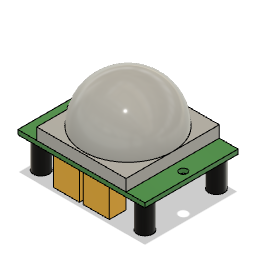
Dectecteur v4 (Autodesk Fusion 360 archive; units mm, degrees)
design "SEN0018_Detecteur UI.R"
Autodesk Fusion 360 part; units mm, degrees
sketch "Esquisse1" plane through (0, 0, 0) normal (0, 1, 0) x (1, 0, 0)
  line L0 (0, 0) -> (32.7, 0)
  line L1 (32.7, 0) -> (32.7, -24)
  line L2 (32.7, -24) -> (0, -24)
  line L3 (0, -24) -> (0, 0)
  dimension "d1" = 32.7
  dimension "d2" = 24
  constraint horizontal L0
  constraint vertical L1
  constraint horizontal L2
  constraint vertical L3
  constraint coincident L0.start L3.end
  measures "d1" distance of L0.start L0.end
  measures "d2" distance of L0.start L2.end
extrude "Extrusion1" add sketch "Esquisse1" along normal blind 1.15 makes body 1
sketch "Esquisse2" plane through (0, 1.15, 0) normal (0, 1, 0) x (-1, 0, 0)
  line L0 (0, 24) -> (-32.7, 24)
  line L1 (-32.7, 24) -> (-32.7, 0)
  line L2 (-32.7, 0) -> (0, 0)
  line L3 (0, 0) -> (0, 24)
  line L4 (-4.85, 0) -> (-27.85, 0)
  line L5 (-27.85, 0) -> (-27.85, 24)
  line L6 (-27.85, 24) -> (-4.85, 24)
  line L7 (-4.85, 24) -> (-4.85, 0)
  dimension "d5" = 23
  constraint horizontal L4
  constraint vertical L5
  constraint horizontal L6
  constraint vertical L7
  constraint coincident L0 L5.end
  constraint coincident L2 L4.start
  constraint midpoint L2 L4
  measures "d5" distance of L4.start L4.end
extrude "Extrusion2" add sketch "Esquisse2" along normal blind 3 separate body contours L0 L2 L4 L5 L6 L7 makes body 2
ref_plane "Plan de construction1" through (16.35, 2.65, 12) normal (0, 0, 1) x (1, 0, 0)
sketch "Esquisse3" plane through (16.35, 2.65, 12) normal (0, 0, 1) x (1, 0, 0)
  arc A0 (0, 13) -> (-11.5, 1.5) centre (0, 1.5) ccw
  line L0 (0, 1.5) -> (0, 13) construction
  line L1 (0, 1.5) -> (-11.5, 1.5) construction
  line L2 (-11.5, 1.5) -> (11.5, 1.5)
  line L3 (0, 13) -> (0, 1.5)
  point P0 (-11.5, 1.5)
  dimension "d8" = 90
  constraint coincident P0 A0.end
  constraint midpoint A0.centre L2
  constraint coincident A0.centre L0.start
  measures "d8" angle of L0 L1
revolve "Révolution1" add sketch "Esquisse3" angle 360 about axis through (16.35, 15.65, 12) along (0, -1, 0) bodies 2
sketch "Esquisse5" plane through (0, 0, 0) normal (0, -1, 0) x (1, 0, 0)
  line L0 (32.7, 24) -> (0, 24)
  line L1 (0, 24) -> (0, 0)
  line L2 (0, 0) -> (32.7, 0)
  line L3 (32.7, 0) -> (32.7, 24)
  circle A0 centre (3, 21) radius 2
  circle A1 centre (29.7, 21) radius 2
  circle A2 centre (29.7, 2.5849) radius 2
  circle A3 centre (3, 2.5849) radius 2
  line L4 (8.3, 23.15) -> (15, 23.15)
  line L5 (15, 23.15) -> (15, 18.85)
  line L6 (15, 18.85) -> (8.3, 18.85)
  line L7 (8.3, 18.85) -> (8.3, 23.15)
  line L8 (16, 23.15) -> (22.7, 23.15)
  line L9 (22.7, 23.15) -> (22.7, 18.85)
  line L10 (22.7, 18.85) -> (16, 18.85)
  line L11 (16, 18.85) -> (16, 23.15)
  line L12 (12.35, 3.7849) -> (20.35, 3.7849)
  line L13 (20.35, 3.7849) -> (20.35, 1.3849)
  line L14 (20.35, 1.3849) -> (12.35, 1.3849)
  line L15 (12.35, 1.3849) -> (12.35, 3.7849)
  line L16 (14.35, 2.8349) -> (14.85, 2.8349)
  line L17 (14.85, 2.8349) -> (14.85, 2.3349)
  line L18 (14.85, 2.3349) -> (14.35, 2.3349)
  line L19 (14.35, 2.3349) -> (14.35, 2.8349)
  line L20 (17.85, 2.8349) -> (18.35, 2.8349)
  line L21 (18.35, 2.8349) -> (18.35, 2.3349)
  line L22 (18.35, 2.3349) -> (17.85, 2.3349)
  line L23 (17.85, 2.3349) -> (17.85, 2.8349)
  line L24 (16.1, 2.8349) -> (16.6, 2.8349)
  line L25 (16.6, 2.8349) -> (16.6, 2.3349)
  line L26 (16.6, 2.3349) -> (16.1, 2.3349)
  line L27 (16.1, 2.3349) -> (16.1, 2.8349)
  line L28 (3, 21) -> (29.7, 21) construction
  line L29 (29.7, 21) -> (29.7, 2.5849) construction
  line L30 (29.7, 2.5849) -> (3, 2.5849) construction
  line L31 (3, 2.5849) -> (3, 21) construction
  line L32 (16.35, 2.3349) -> (16.35, 1.3849) construction
  line L33 (16.35, 1.3849) -> (16.35, 0) construction
  line L34 (18.35, 2.5849) -> (20.35, 2.5849) construction
  dimension "d10" = 4
  dimension "d11" = 4
  dimension "d12" = 4
  dimension "d13" = 4
  dimension "d14" = 3
  dimension "d15" = 3
  dimension "d16" = 3
  dimension "d17" = 2.5849
  dimension "d18" = 6.7
  dimension "d19" = 4.3
  dimension "d20" = 1
  dimension "d21" = 2.15
  dimension "d22" = 7
  dimension "d23" = 8
  dimension "d24" = 0.5
  dimension "d25" = 0.5
  dimension "d26" = 2
  dimension "d27" = 2
  dimension "d29" = 2.4
  constraint horizontal L4
  constraint vertical L5
  constraint horizontal L6
  constraint vertical L7
  constraint horizontal L8
  constraint vertical L9
  constraint horizontal L10
  constraint vertical L11
  constraint horizontal L12
  constraint vertical L13
  constraint horizontal L14
  constraint vertical L15
  constraint horizontal L16
  constraint vertical L17
  constraint horizontal L18
  constraint vertical L19
  constraint horizontal L20
  constraint vertical L21
  constraint horizontal L22
  constraint vertical L23
  constraint horizontal L24
  constraint vertical L25
  constraint horizontal L26
  constraint vertical L27
  constraint horizontal L28
  constraint vertical L29
  constraint horizontal L30
  constraint vertical L31
  constraint coincident A0.centre L28.start
  constraint coincident A1.centre L28.end
  constraint coincident A2.centre L29.end
  constraint coincident A3.centre L30.end
  constraint equal L6 L10
  constraint equal L5 L11
  constraint collinear L4 L8
  constraint equal L16 L20
  constraint equal L20 L23
  constraint equal L21 L27
  constraint equal L24 L27
  constraint collinear L16 L24
  constraint collinear L20 L24
  constraint midpoint L26 L32.start
  constraint coincident L14 L32.end
  constraint midpoint L14 L32.end
  constraint vertical L32
  constraint coincident L2 L33.end
  constraint midpoint L2 L33.end
  constraint vertical L33
  constraint midpoint L21 L34.start
  constraint midpoint L13 L34.end
  constraint horizontal L34
  constraint coincident L30 L34.end
  measures "d10" diameter of A0
  measures "d11" diameter of A1
  measures "d12" diameter of A2
  measures "d13" diameter of A3
  measures "d14" distance of L0 A0.centre
  measures "d15" distance of L1 A0.centre
  measures "d16" distance of L3 L29
  measures "d17" distance of L2 L30
  measures "d18" distance of L5.end L6.end
  measures "d19" distance of L4.start L6.end
  measures "d20" distance of L5 L11
  measures "d21" distance of L8 L28
  measures "d22" distance of A1.centre L9
  measures "d23" distance of L12.start L12.end
  measures "d24" distance of L16.start L16.end
  measures "d25" distance of L16.start L18.end
  measures "d26" distance of L15 L18.end
  measures "d27" distance of L13 L21.end
  measures "d29" distance of L12.end L13.end
extrude "Extrusion3" add sketch "Esquisse5" along normal blind 7.8 separate body contours A0 | A1 | A2 | A3 makes body 3 at (4.9901, -5.2, 2.3857) makes body 4 at (31.6901, -5.2, 20.8009) makes body 5 at (4.9901, -5.2, 20.8009) makes body 6 at (31.6901, -5.2, 2.3857)
extrude "Extrusion4" add sketch "Esquisse5" along normal blind 8 separate body contours L4 L5 L6 L7 | L8 L9 L10 L11 makes body 7 at (10.5333, -2.6667, 23.15) makes body 8 at (20.4667, -2.6667, 18.85)
extrude "Extrusion5" add sketch "Esquisse5" along normal blind 8.3 separate body contours L16 L17 L18 L19 | L20 L21 L22 L23 | L24 L25 L26 L27 makes body 9 at (14.5167, -2.7667, 2.8349) makes body 10 at (16.2667, -2.7667, 2.8349) makes body 11 at (17.85, -2.7667, 2.5016)
extrude "Extrusion6" add sketch "Esquisse5" along normal blind 2 separate body contours L12 L13 L14 L15 makes body 12
sketch "Esquisse6" plane through (0, 1.15, 0) normal (0, 1, 0) x (-1, 0, 0)
  line L0 (0, 24) -> (-32.7, 24)
  line L1 (-32.7, 24) -> (-32.7, 0)
  line L2 (-32.7, 0) -> (0, 0)
  line L3 (0, 0) -> (0, 24)
  circle A0 centre (-30.6, 12) radius 1
  line L4 (-32.7, 12) -> (0, 12) construction
  circle A1 centre (-2.1, 12) radius 1
  dimension "d38" = 2
  dimension "d39" = 2.1
  dimension "d40" = 2
  dimension "d41" = 2.1
  constraint midpoint L1 L4.start
  constraint midpoint L3 L4.end
  constraint coincident A0.centre L4
  constraint coincident L4 A1.centre
  measures "d38" diameter of A0
  measures "d39" distance of L1 A0.centre
  measures "d40" diameter of A1
  measures "d41" distance of L3 A1.centre
extrude "Extrusion7" cut sketch "Esquisse6" against normal up to surface (1.15 mm away) contours A0 | A1 bodies 1
equation "d16 = d15"
equation "d21 = d19 / 2"
equation "d27 = d26"
equation "d40 = d38"
equation "d41 = d39"

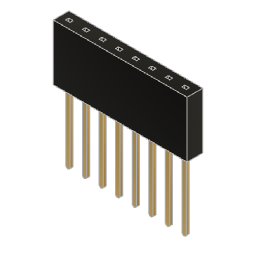
design "Barette_male_femelle_wemos"
Autodesk Fusion 360 part; units mm, degrees
sketch "Esquisse1" plane through (0, 0, 0) normal (0, 0, 1) x (1, 0, 0)
  line L0 (10.25, -1.2) -> (-10.25, -1.2)
  line L1 (-10.25, -1.2) -> (-10.25, 1.2)
  line L2 (-10.25, 1.2) -> (10.25, 1.2)
  line L3 (10.25, 1.2) -> (10.25, -1.2)
  line L4 (10.25, -1.2) -> (-10.25, 1.2) construction
  line L5 (-10.25, -1.2) -> (10.25, 1.2) construction
  line L6 (-9.2988, 0.225) -> (-8.6388, 0.225)
  line L7 (-8.6387, 0.225) -> (-8.6387, -0.225)
  line L8 (-8.6387, -0.225) -> (-9.2988, -0.225)
  line L9 (-9.2988, -0.225) -> (-9.2988, 0.225)
  dimension "d1" = 20.5
  dimension "d2" = 2.4
  dimension "d3" = 0.66
  dimension "d4" = 0.45
  dimension "d5" = 0.225
  dimension "d6" = 0.9513
  constraint horizontal L0
  constraint perpendicular L0 L1
  constraint parallel L0 L2
  constraint parallel L1 L3
  constraint coincident L4 origin
  constraint coincident L5 origin
  constraint horizontal L6
  constraint vertical L7
  constraint horizontal L8
  constraint vertical L9
  measures "d1" distance of L1.end L2.end
  measures "d2" distance of L0.end L1.end
  measures "d3" distance of L6.start L7.start
  measures "d4" distance of L6.start L8.end
  measures "d5" distance of origin L6
  measures "d6" distance of L1 L9
extrude "Extrusion1" add sketch "Esquisse1" along normal blind 8.6 contours L0 L1 L2 L3 | L6 L7 L8 L9 makes body 1
extrude "Extrusion2" add sketch "Esquisse1" against normal blind 11 separate body contours L6 L7 L8 L9 makes body 2
extrude "Extrusion3" cut sketch "Esquisse1" along normal up to surface (8.6 mm away) contours L6 L7 L8 L9 bodies 1
chamfer "Chanfrein1" distance 0.2 angle 45 2 edges at (-8.6387, 0, -11) (-9.2988, 0, -11) on bodies 2
pattern_linear "Réseau R1" count 8 spacing 2.54 along (1, 0, 0) of "Extrusion3"
pattern_linear "Réseau R2" count 8 spacing 2.54 along (1, 0, 0) of bodies 2 makes body 3 at (-6.5388, -0.225, -7.2) makes body 4 at (-3.9988, -0.225, -7.2) makes body 5 at (-1.4588, -0.225, -7.2) makes body 6 at (1.0812, -0.225, -7.2) makes body 7 at (3.6212, -0.225, -7.2) makes body 8 at (6.3812, 0.225, -7.2) makes body 9 at (8.7013, -0.225, -7.2)
equation "d5 = d4 / 2"
equation "d6 = ( d1 - 8 * d3 ) / 16"
named bodies: "Corps", "Pin", "Pin (1)", "Pin (2)", "Pin (3)", "Pin (4)", "Pin (5)", "Pin (6)", "Pin (7)"
